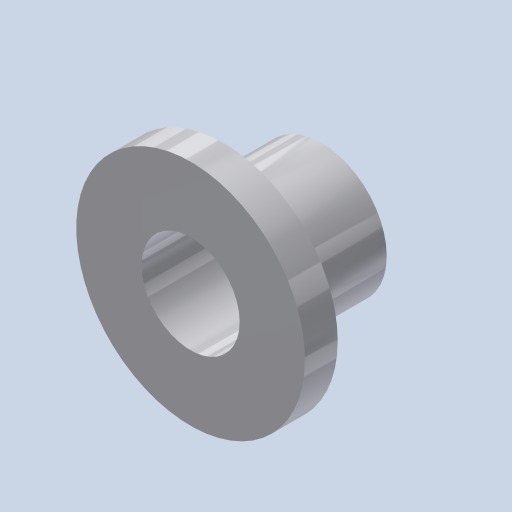
# Autodesk Inventor part: D3040-7130B
Saved by Autodesk Inventor 2023 (Build 270158000, 158)
## iProperties
Created: 2015-11-28
Part Number: D3040-7130B
Material: アセタール樹脂、白
Document SubType Name: Modeling
Designer: hiroaki
Density: 1.425 g/cm^3
Appearance: 積雪
Mass: 0.0682707 g
Surface Area: 1.60221 cm^2
Volume: 0.0479093 cm^3
Author: hiroaki
Autodesk Inventor part; units mm, degrees
ref_plane "YZ Plane" through (0, 0, 0) normal (1, 0, 0) x (0, 1, 0)
ref_plane "XZ Plane" through (0, 0, 0) normal (0, 1, 0) x (-1, 0, 0)
ref_plane "XY Plane" through (0, 0, 0) normal (0, 0, 1) x (1, 0, 0)
sketch "スケッチ1" plane through (0, 0, 0) normal (0, 0, 1) x (1, 0, 0)
  line L0 (0, 0) -> (0, 1.2478) construction
  line L1 (1.5, 2) -> (1.5, -2)
  line L2 (1.5, -2) -> (3.5, -2)
  line L3 (3.5, -2) -> (3.5, -1)
  line L4 (3.5, -1) -> (2, -1)
  line L5 (2, -1) -> (2, 2)
  line L6 (2, 2) -> (1.5, 2)
  point P0 (1.5, 0)
  dimension "d0" = 1.5
  dimension "d1" = 2
  dimension "d2" = 3
  dimension "d3" = 1
  dimension "d4" = 3.5
  constraints: 14 end point, 5 perpendicular, 2 vertical, 1 horizontal alignment, 1 midpoint
  measures "d0" distance between parallel lines of L0 L1
  measures "d1" distance between parallel lines of L0 L5
  measures "d2" distance between parallel lines of L4 L6
  measures "d3" distance of L2.end L3.end
  measures "d4" distance between parallel lines of L3 L0
revolve "回転1" add sketch "スケッチ1" angle 360 about axis through (0, 0, 0) along (0, 1, 0)
